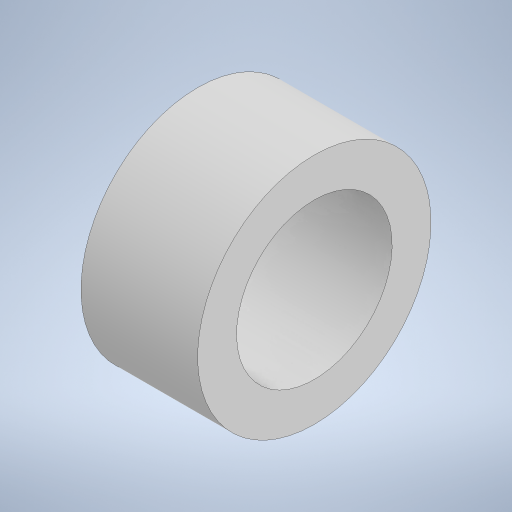
# Autodesk Inventor part: DNM pin 12x6x40 spacer.STEP
Saved by Autodesk Inventor 2023 (Build 270158000, 158)
## iProperties
Created: 2022-03-31
Part Number: DNM pin 12x6x40 spacer.STEP
Material: Generic
Document SubType Name: Modeling
Designer: Zain Ali
Density: 1 g/cm^3
Appearance: Default
Author: Zain Ali
Autodesk Inventor part; units mm, degrees
ref_plane "YZ Plane" through (0, 0, 0) normal (1, 0, 0) x (0, 1, 0)
ref_plane "XZ Plane" through (0, 0, 0) normal (0, 1, 0) x (-1, 0, 0)
ref_plane "XY Plane" through (0, 0, 0) normal (0, 0, 1) x (1, 0, 0)
sketch "Sketch2" plane through (0, 0, 0) normal (1, 0, 0) x (0, 1, 0)
  circle A0 centre (0, 0) radius 9
  circle A1 centre (0, 0) radius 6
  dimension "d2" = 18
  dimension "d3" = 12
  constraints: 2 centre point, 2 coincident
  measures "d2" diameter of A0
  measures "d3" diameter of A1
extrude "Extrusion1" add sketch "Sketch2" along normal blind 9
body "Solid2"
